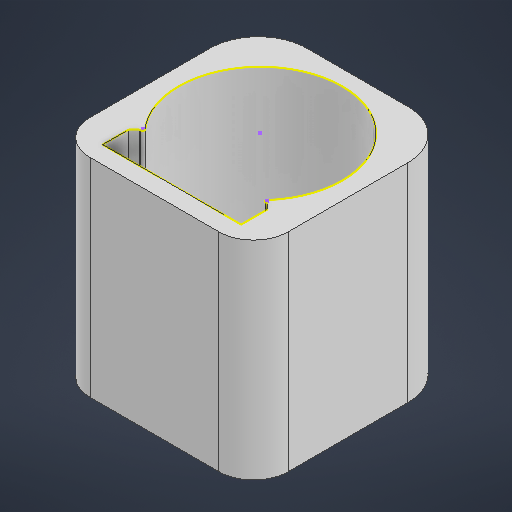
# Autodesk Inventor part: mount
Saved by Autodesk Inventor 2026.1 (Build 301233020, 233B)
## iProperties
Created: 2025-12-18
Part Number: mount
Material: Generic
Document SubType Name: Modeling
Designer: Fish
Density: 1 g/cm^3
Appearance: Default
Author: Fish
Autodesk Inventor part; units mm, degrees
ref_plane "YZ Plane" through (0, 0, 0) normal (1, 0, 0) x (0, 1, 0)
ref_plane "XZ Plane" through (0, 0, 0) normal (0, 1, 0) x (-1, 0, 0)
ref_plane "XY Plane" through (0, 0, 0) normal (0, 0, 1) x (1, 0, 0)
sketch "Sketch1" plane through (0, 0, 0) normal (0, 1, 0) x (-1, 0, 0)
  circle A0 centre (0, 0) radius 11.5
  circle A1 centre (0, 0) radius 11.8
  line L0 (10, 12.5) -> (-10, 12.5)
  line L1 (-10, 12.5) -> (-10, 8.2614)
  line L2 (-10, 8.2614) -> (10, 8.2614)
  line L3 (10, 8.2614) -> (10, 12.5)
  line L4 (10, 12.5) -> (-10, 8.2614) construction
  line L5 (-10, 12.5) -> (10, 8.2614) construction
  line L6 (0, 10.3807) -> (0, -11.5) construction
  line L7 (10, 12.5) -> (-10, 12.5)
  line L8 (-10, 12.5) -> (-10, 12.8)
  line L9 (-10, 12.8) -> (10, 12.8)
  line L10 (10, 12.8) -> (10, 12.5)
  line L11 (-14.3, 15.3) -> (14.3, 15.3)
  line L12 (14.3, 15.3) -> (14.3, -14)
  line L13 (14.3, -14) -> (-14.3, -14)
  line L14 (-14.3, -14) -> (-14.3, 15.3)
  point P0 (8, 8.2614)
  point P1 (-8, 8.2614)
  point P2 (0, -14)
  point P3 (8.4256, 8.2614)
  point P4 (-8.4256, 8.2614)
  dimension "d0" = 23
  dimension "d1" = 0.3
  dimension "d2" = 24
  dimension "d3" = 16
  dimension "d4" = 20
  dimension "d5" = 0.3
  dimension "d6" = 2.5
  dimension "d7" = 2.5
  dimension "d8" = 2.5
  dimension "d9" = 14.3
  dimension "d10" = 14.3
  constraints: 30 end point, 6 parallel, 3 horizontal, 3 midpoint, 3 perpendicular, 3 point on circle, 3 point on line, 2 centre point, 2 coincident, 1 vertical
  measures "d0" diameter of A0
  measures "d1" radial gap between concentric circles of A1 A0
  measures "d2" distance from line of L0 L6.end
  measures "d3" distance of point (-8, 8.261) A0.end
  measures "d4" distance of L0.start L0.end
  measures "d5" distance between parallel lines of L9 L0
  measures "d6" distance between parallel lines of L11 L9
  measures "d7" distance of point (0, -14) L6.end
  measures "d8" distance edge to line of A1 L14
  measures "d9" distance between parallel lines of L14 L6
  measures "d10" distance between parallel lines of L12 L6
extrude "Extrusion1" add sketch "Sketch1" along normal blind 30
fillet "Fillet1" radius 0.25 2 edges at (8.4256, 15, 8.2614) (-8.4256, 15, 8.2614)
chamfer "Chamfer1" distance 0.75 angle 45 2 edges at (-10, 15, 8.2614) (10, 15, 8.2614)
sketch "Sketch2" plane through (14.3, 0, -14) normal (0, 0, -1) x (-1, 0, 0)
  line L0 (2.5, 30) -> (26.1, 30) projected
  line L1 (2.5, 30) -> (26.1, 30)
  line L2 (26.1, 30) -> (26.1, 0)
  line L3 (26.1, 0) -> (2.5, 0)
  line L4 (2.5, 0) -> (2.5, 30)
  line L5 (0, 0) -> (28.6, 0) projected
  circle A0 centre (6.3, 2.3324) radius 3.5
  circle A1 centre (6.3, 2.3324) radius 3.8
  line L6 (3.3, 0) -> (9.3, 0) construction
  line L7 (2.8, 0) -> (2.8, 30)
  point P0 (14.3, 0)
  point P1 (23.1144, 30)
  point P2 (5.4856, 30)
  point P3 (2.5, 2.3324)
  point P4 (3.6904, 0)
  point P5 (9.3, 0)
  point P6 (2.5, 2.3324)
  point P7 (2.5, 0.8525)
  point P8 (8.9096, 0)
  dimension "d17" = 7
  dimension "d18" = 0.3
  dimension "d20" = 6
  dimension "d25" = 0.3
  constraints: 12 end point, 4 point on line, 2 centre point, 2 horizontal, 2 parallel, 2 perpendicular, 2 point on circle, 1 coincident, 1 tangent
  measures "d17" diameter of A0
  measures "d18" radial gap between concentric circles of A1 A0
  measures "d20" distance of L6.end L6.start
  measures "d25" distance between parallel lines of L4 L7
extrude "Extrusion2" cut sketch "Sketch2" against normal up to surface contours A1 L7 | A1 L3 A0 L7 | L7 A0 L3 A1 | A0 L3 | L3 A0 A1 | L3 A0
fillet "Fillet2" radius 0.25 2 edges at (5, 0, -12.3442) (11, 0, -9.1354)
sketch "Sketch4" plane through (14.3, 30, -14) normal (0, 0, -1) x (-1, 0, 0)
  arc A0 (2.8264, -30) -> (3.0408, -29.6215) centre (2.8264, -29.75) ccw projected
  arc A1 (9.5592, -29.6215) -> (3.0408, -29.6215) centre (6.3, -27.6676) ccw projected
  arc A2 (9.5592, -29.6215) -> (9.7736, -30) centre (9.7736, -29.75) ccw projected
  line L0 (9.7736, -30) -> (28.6, -30) projected
  line L1 (28.6, -30) -> (28.6, 0) projected
  line L2 (0, 0) -> (28.6, 0) projected
  line L3 (0, -30) -> (0, 0) projected
  line L4 (0, -30) -> (2.8264, -30) projected
  line L5 (3.0764, -29.0955) -> (9.5236, -29.0955)
  line L6 (9.5236, -29.0955) -> (9.5236, -29.986)
  line L7 (9.5236, -29.986) -> (3.0764, -29.986)
  line L8 (3.0764, -29.986) -> (3.0764, -29.0955)
  arc A3 (9.5592, -29.6215) -> (9.7736, -30) centre (9.7736, -29.75) ccw projected
  point P0 (14.3, -30)
  dimension "d26" = 6.4473
  constraints: 8 end point, 2 parallel, 2 tangent, 1 horizontal, 1 perpendicular
  measures "d26" distance of L5.start L5.end
fillet "Fillet3" radius 7 2 edges at (14.3, 15, -14) (-14.3, 15, -14)
fillet "Fillet4" radius 5 2 edges at (-14.3, 15, 15.3) (14.3, 15, 15.3)
sketch "Sketch5" plane through (0, 30, 0) normal (0, 1, 0) x (1, 0, 0)
  arc A0 (8.8144, -7.8451) -> (-8.8144, -7.8451) centre (0, 0) ccw projected
  line L0 (10, -12.8) -> (-10, -12.8) projected
  line L1 (-10, -12.8) -> (-10, -9.0114) projected
  line L2 (-9.25, -8.2614) -> (-10, -9.0114) projected
  line L3 (-9.25, -8.2614) -> (-9.0011, -8.2614) projected
  arc A1 (-9.0011, -8.2614) -> (-8.8144, -7.8451) centre (-9.0011, -8.0114) ccw projected
  line L4 (10, -9.0114) -> (10, -12.8) projected
  arc A2 (-9.0011, -8.2614) -> (-8.8144, -7.8451) centre (-9.0011, -8.0114) ccw projected
  arc A3 (8.8144, -7.8451) -> (-8.8144, -7.8451) centre (0, 0) ccw projected
  arc A4 (8.8144, -7.8451) -> (9.0011, -8.2614) centre (9.0011, -8.0114) ccw projected
  line L5 (9.0011, -8.2614) -> (9.25, -8.2614) projected
  line L6 (10, -9.0114) -> (9.25, -8.2614) projected
  line L7 (10, -9.0114) -> (10, -12.8) projected
  line L8 (10, -12.8) -> (-10, -12.8) projected
  line L9 (-10, -12.8) -> (-10, -9.0114) projected
  line L10 (-9.25, -8.2614) -> (-10, -9.0114) projected
  line L11 (-9.25, -8.2614) -> (-9.0011, -8.2614) projected
  constraints: 3 centre point
equation "\"d10\" = d9"
body "Solid1"
